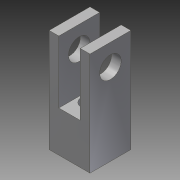
# Autodesk Inventor part: piston_rod_connector
Saved by Autodesk Inventor 2015 (Build 190159000, 159)
## iProperties
Created: 2017-02-22
Part Number: piston_rod_connector
Material: Steel, Non-Alloy
Document SubType Name: Modeling
Designer: Guy
Density: 7.85 g/cm^3
Appearance: Steel
Author: Guy
Autodesk Inventor part; units mm, degrees
ref_plane "YZ Plane" through (0, 0, 0) normal (1, 0, 0) x (0, 1, 0)
ref_plane "XZ Plane" through (0, 0, 0) normal (0, 1, 0) x (-1, 0, 0)
ref_plane "XY Plane" through (0, 0, 0) normal (0, 0, 1) x (1, 0, 0)
sketch "Sketch1" plane through (0, 0, 0) normal (0, 0, 1) x (1, 0, 0)
  line L0 (0, 0) -> (9.5, 0)
  line L1 (9.5, 0) -> (9.5, 9.5)
  line L2 (9.5, 9.5) -> (0, 9.5)
  line L3 (0, 9.5) -> (0, 0)
  dimension "d0" = 9.5
  dimension "d1" = 9.5
  constraints: 8 end point, 2 parallel, 1 horizontal, 1 perpendicular
  measures "d0" distance of L2.end L1.end
  measures "d1" distance of L1.end L0.end
extrude "Extrusion1" add sketch "Sketch1" along normal blind 24
sketch "Sketch2" plane through (0, 9.5, 0) normal (0, 1, 0) x (1, 0, 0)
  line L0 (0, -24) -> (9.5, -24) projected
  line L1 (2.25, -24) -> (7.25, -24)
  line L2 (7.25, -24) -> (7.25, -9.5)
  line L3 (7.25, -9.5) -> (2.25, -9.5)
  line L4 (2.25, -9.5) -> (2.25, -24)
  line L5 (0, 0) -> (0, -24) projected
  dimension "d4" = 14.5
  dimension "d5" = 5
  dimension "d6" = 2.25
  constraints: 8 end point, 2 parallel, 1 horizontal, 1 perpendicular, 1 point on line
  measures "d4" distance of L3.end L1.start
  measures "d5" distance between parallel lines of L2 L4
  measures "d6" distance between parallel lines of L5 L4
extrude "Extrusion2" cut sketch "Sketch2" against normal up to next
sketch "Sketch3" plane through (9.5, 0, 0) normal (1, 0, 0) x (0, 0, -1)
  circle A0 centre (-19, 4.75) radius 2.5
  line L0 (-24, 0) -> (-24, 9.5) projected
  line L1 (0, 9.5) -> (-24, 9.5) projected
  point P0 (0, 0)
  dimension "d9" = 5
  dimension "d10" = 5
  dimension "d11" = 4.75
  constraints: 1 centre point
  measures "d9" diameter of A0
  measures "d10" distance from line of L0 A0.centre
  measures "d11" distance from line of A0.centre L1
extrude "Extrusion3" cut sketch "Sketch3" against normal through all
sketch "Sketch4" plane through (2.25, 9.5, 9.5) normal (0, 0, 1) x (1, 0, 0)
  circle A0 centre (2.5, -4.75) radius 2
  line L0 (0, 0) -> (5, 0) projected
  line L1 (0, -9.5) -> (0, 0) projected
  point P0 (-2.25, -9.5)
  dimension "d14" = 4
  dimension "d15" = 4.75
  dimension "d16" = 2.5
  constraints: 1 centre point
  measures "d14" diameter of A0
  measures "d15" distance from line of A0.centre L0
  measures "d16" distance from line of L1 A0.centre
extrude "Extrusion4" cut sketch "Sketch4" against normal up to next
body "Solid1"
